Autodesk Inventor part; units mm, degrees
(part 2 of 2)
  point P64 (-30.0868, -25.5338)
  point P65 (-28.4719, -25.5695)
  point P66 (-28.5952, -25.7916)
  point P67 (-29.6277, -25.9647)
  point P68 (-29.8066, -26.1693)
  point P69 (-30.1253, -26.3527)
  point P70 (-30.5749, -26.3003)
  point P71 (-30.9459, -26.7717)
  point P72 (-31.5299, -27.0871)
  point P73 (-32.0372, -27.182)
  point P74 (-32.5042, -26.99)
  point P75 (-32.8272, -27.3923)
  point P76 (-33.4531, -27.6243)
  point P77 (-34.2071, -27.4345)
  point P78 (-31.7361, -19.9483)
  point P79 (-29.2525, -20.4913)
  point P80 (-32.0372, -20.4201)
  point P81 (-30.3205, -21.1678)
  point P82 (-29.021, -21.4527)
  point P83 (-26.9113, -22.7987)
  point P84 (-35.5982, -27.4344)
  point P85 (-34.8583, -27.8265)
  point P86 (-33.4197, -28.03)
  point P87 (-32.891, -28.5179)
  point P88 (-32.247, -29.4023)
  point P89 (-31.0508, -30.3327)
  point P90 (-30.1511, -30.409)
  point P91 (-29.5919, -30.9021)
  point P92 (-30.1816, -31.0393)
  point P93 (-30.5749, -30.8665)
  point P94 (-30.9459, -31.2172)
  point P95 (-30.9245, -31.6466)
  point P96 (-30.7152, -32.3776)
  point P97 (-30.4644, -32.8075)
  point P98 (-30.4929, -33.1442)
  point P99 (-30.4301, -33.5894)
  point P100 (-29.682, -34.4672)
  point P101 (-30.3043, -34.2354)
  point P102 (-30.7153, -34.2083)
  point P103 (-31.313, -34.2745)
  point P104 (-31.7361, -34.5229)
  point P105 (-32.8272, -35.1172)
  point P106 (-32.7063, -34.6795)
  point P107 (-32.2108, -34.2055)
  point P108 (-32.4143, -34.1566)
  point P109 (-32.891, -34.3372)
  point P110 (-33.6445, -34.4152)
  point P111 (-33.5082, -34.1401)
  point P112 (-32.9457, -34.0685)
  point P113 (-32.6446, -33.8759)
  point P114 (-32.9346, -33.6943)
  point P115 (-33.3611, -33.5127)
  point P116 (-32.891, -33.3167)
  point P117 (-32.4284, -33.3696)
  point P118 (-31.9001, -33.5402)
  point P119 (-31.4764, -33.6887)
  point P120 (-31.1352, -33.1443)
  point P121 (-31.1855, -32.719)
  point P122 (-31.367, -32.1247)
  point P123 (-31.9981, -30.6568)
  point P124 (-32.891, -29.6261)
  point P125 (-33.3321, -29.0765)
  point P126 (-34.1278, -28.6998)
  point P127 (-35.9677, -27.5912)
  point P128 (-32.233, -28.3647)
  point P129 (-31.6958, -28.9797)
  point P130 (-29.3949, -29.4483)
  point P131 (-27.5365, -29.4558)
  point P132 (-32.4284, -28.6281)
  point P133 (-31.4301, -29.4557)
  point P134 (-29.5919, -30.2319)
  point P135 (-31.4058, -28.1532)
  point P136 (-30.3206, -28.5178)
  point P137 (-31.9002, -28.0887)
  point P138 (-30.6071, -28.8216)
  point P139 (-27.2215, -28.3648)
  point P140 (-26.4725, -28.3648)
  point P141 (-30.4031, -27.5183)
  point P142 (-29.8876, -27.6743)
  point P143 (-28.3379, -27.7354)
  point P144 (-27.1102, -27.7354)
  point P145 (-27.1102, -27.9931)
  point P146 (-27.3781, -28.0888)
  point P147 (-28.209, -28.1152)
  point P148 (-29.5156, -28.03)
  point P149 (-30.4929, -27.7354)
  point P150 (-28.4719, -27.1155)
  point P151 (-27.2816, -26.5279)
  point P152 (-26.8336, -26.8291)
  point P153 (-26.3626, -27.4166)
  point P154 (-26.5866, -27.5913)
  point P155 (-26.9113, -27.3623)
  point P156 (-27.3781, -27.182)
  point P157 (-28.8439, -27.5183)
  point P158 (-25.5596, -26.7717)
  point P159 (-25.4467, -26.652)
  point P160 (-27.2215, -25.7437)
  point P161 (-29.049, -26.7161)
  point P162 (-24.6062, -25.9647)
  point P163 (-23.9263, -26.1693)
  point P164 (-22.5249, -26.9237)
  point P165 (-22.1087, -27.182)
  point P166 (-22.1781, -26.9307)
  point P167 (-23.3297, -25.7437)
  point P168 (-24.8837, -24.6744)
  point P169 (-22.3856, -28.5179)
  point P170 (-20.4794, -30.5023)
  point P171 (-23.7992, -26.652)
  point P172 (-22.5893, -27.182)
  point P173 (-20.9573, -29.3205)
  point P174 (-20.3852, -29.9489)
  point P175 (-19.466, -30.5023)
  point P176 (-18.6876, -30.5717)
  point P177 (-21.1885, -30.5716)
  point P178 (-21.3807, -30.8665)
  point P179 (-21.8293, -31.0393)
  point P180 (-22.0581, -30.5023)
  point P181 (-22.5249, -29.7113)
  point P182 (-23.1291, -28.6998)
  point P183 (-23.4495, -28.8216)
  point P184 (-22.2686, -31.2955)
  point P185 (-24.4126, -35.4531)
  point P186 (-24.4242, -35.2548)
  point P187 (-24.0393, -35.0098)
  point P188 (-22.8145, -33.0852)
  point P189 (-23.4098, -29.3205)
  point P190 (-24.4242, -28.1152)
  point P191 (-23.5497, -32.1868)
  point P192 (-24.8836, -33.0853)
  point P193 (-25.7863, -32.5427)
  point P194 (-25.5918, -32.4133)
  point P195 (-24.2648, -31.7834)
  point P196 (-23.9962, -30.5022)
  point P197 (-24.3657, -28.8218)
  point P198 (-25.1447, -27.6244)
  point P199 (-25.2341, -28.7674)
  constraints: 1 centre point, 1 point on line, 1163 other
body "Solid1"
